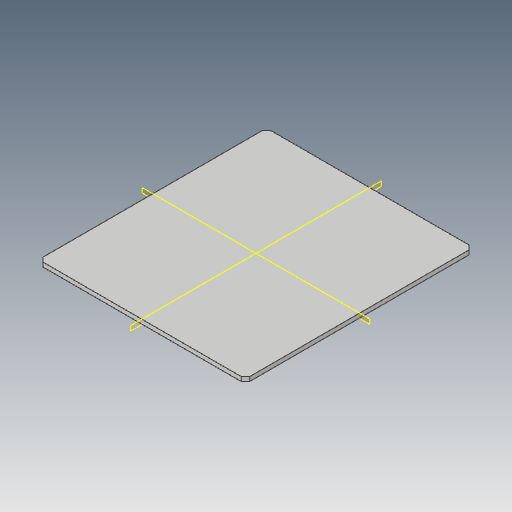
# Autodesk Inventor part: Battery Base Plate
Saved by Autodesk Inventor 2017 (Build 210142000, 142)
## iProperties
Created: 2019-01-21
Part Number: Battery Base Plate
Material: Generic
Document SubType Name: Modeling
Designer: jb0839
Density: 1 g/cm^3
Appearance: Default
Mass: 84.6238 g
Surface Area: 553.593 cm^2
Volume: 84.6238 cm^3
Author: jb0839
Autodesk Inventor part; units mm, degrees
ref_plane "YZ Plane" through (0, 0, 0) normal (1, 0, 0) x (0, 1, 0)
ref_plane "XZ Plane" through (0, 0, 0) normal (0, 1, 0) x (-1, 0, 0)
ref_plane "XY Plane" through (0, 0, 0) normal (0, 0, 1) x (1, 0, 0)
sketch "Sketch1" plane through (0, 0, 0) normal (0, 1, 0) x (-1, 0, 0)
  line L0 (0, 0) -> (155.575, 0)
  line L1 (155.575, 0) -> (155.575, -171.45)
  line L2 (155.575, -171.45) -> (0, -171.45)
  line L3 (0, -171.45) -> (0, 0)
  dimension "d0" = 155.575
  dimension "d1" = 171.45
  constraints: 8 end point, 2 parallel, 1 horizontal, 1 perpendicular
  measures "d0" distance of L1.end L2.end
  measures "d1" distance of L0.end L1.end
extrude "Extrusion1" add sketch "Sketch1" along normal blind 3.175
chamfer "Chamfer1" distance 3.175 angle 45 4 edges at (0, 1.5875, 0) (-155.575, 1.5875, 0) (-155.575, 1.5875, -171.45) (0, 1.5875, -171.45)
ref_plane "Work Plane1" through (-77.7875, 0, -3.175) normal (1, 0, 0) x (0, 0, -1)
ref_plane "Work Plane2" through (-152.4, 0, -85.725) normal (0, 0, 1) x (1, 0, 0)
body "Solid1"
